Autodesk Fusion 360 part; units mm, degrees
(part 2 of 2)
sketch "Sketch1" plane through (0, 0, 0) normal (0, 0, 1) x (1, 0, 0)
  line L0 (8.5, 0) -> (91.5, 0)
  line L1 (100, 8.5) -> (100, 91.5)
  line L2 (91.5, 100) -> (8.5, 100)
  line L3 (0, 91.5) -> (0, 8.5)
  line L4 (8.5, 100) -> (8.5, 91.5)
  line L5 (8.5, 91.5) -> (0, 91.5)
  line L6 (91.5, 100) -> (91.5, 91.5)
  line L7 (91.5, 91.5) -> (100, 91.5)
  line L8 (8.5, 0) -> (8.5, 8.5)
  line L9 (8.5, 8.5) -> (0, 8.5)
  line L10 (91.5, 0) -> (91.5, 8.5)
  line L11 (91.5, 8.5) -> (100, 8.5)
  circle A0 centre (28.5, 95.75) radius 1.465
  circle A1 centre (71.5, 95.75) radius 1.465
  circle A2 centre (28.5, 4.25) radius 1.465
  circle A3 centre (71.5, 4.25) radius 1.465
  dimension "d11" = 8.5
  dimension "d12" = 8.5
  dimension "d13" = 8.5
  dimension "d14" = 8.5
  dimension "d15" = 8.5
  dimension "d16" = 8.5
  dimension "d17" = 83
  dimension "d18" = 83
  dimension "d19" = 8.5
  dimension "d20" = 8.5
  dimension "d21" = 8.5
  dimension "d22" = 8.5
  dimension "d25" = 2.93
  dimension "d26" = 4.25
  dimension "d27" = 20
  dimension "d28" = 2.93
  dimension "d29" = 4.25
  dimension "d30" = 20
  dimension "d31" = 2.93
  dimension "d32" = 4.25
  dimension "d33" = 20
  dimension "d34" = 2.93
  dimension "d35" = 4.25
  dimension "d36" = 20
  constraint horizontal L0
  constraint vertical L1
  constraint horizontal L2
  constraint vertical L3
  constraint vertical L4
  constraint horizontal L5
  constraint vertical L6
  constraint horizontal L7
  constraint vertical L8
  constraint horizontal L9
  constraint vertical L10
  constraint horizontal L11
  measures "d11" distance of L10.end L1.start
  measures "d12" distance of L0.end L10.end
  measures "d13" distance of L2.start L6.end
  measures "d14" distance of L6.end L1.end
  measures "d15" distance of L2.end L4.end
  measures "d16" distance of L4.end L3.start
  measures "d17" distance of L3.start L3.end
  measures "d18" distance of L0.start L0.end
  measures "d19" distance of L0.start L8.end
  measures "d20" distance of L8.end L3.end
  measures "d21" distance of origin L0.start
  measures "d22" distance of origin L9
  measures "d25" diameter of A0
  measures "d26" distance of L2 A0.centre
  measures "d27" distance of L4 A0.centre
  measures "d28" diameter of A1
  measures "d29" distance of L2 A1.centre
  measures "d30" distance of L6 A1.centre
  measures "d31" diameter of A2
  measures "d32" distance of L0 A2.centre
  measures "d33" distance of L8 A2.centre
  measures "d34" diameter of A3
  measures "d35" distance of L0 A3.centre
  measures "d36" distance of L10 A3.centre
extrude "Extrude1" add sketch "Sketch1" along normal blind 2

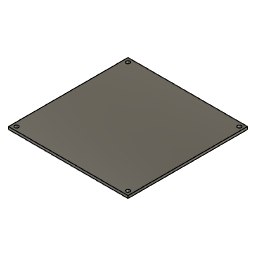
design "подставка"
Autodesk Fusion 360 part; units mm, degrees
sketch "Sketch1" plane through (0, 0, 0) normal (0, 0, 1) x (1, 0, 0)
  line L0 (0, 0) -> (96, 0)
  line L1 (96, 0) -> (96, 96)
  line L2 (96, 96) -> (0, 96)
  line L3 (0, 96) -> (0, 0)
  dimension "d1" = 96
  dimension "d2" = 96
  constraint horizontal L0
  constraint vertical L1
  constraint horizontal L2
  constraint vertical L3
  constraint coincident L0.start L3.end
  measures "d1" distance of L0.start L0.end
  measures "d2" distance of L0.start L2.end
extrude "Extrude1" add sketch "Sketch1" along normal blind 2
sketch "Sketch2" plane through (0, 0, 2) normal (0, 0, 1) x (-1, 0, 0)
  line L0 (0, -96) -> (0, 0)
  line L1 (0, 0) -> (-96, 0)
  line L2 (-96, 0) -> (-96, -96)
  line L3 (-96, -96) -> (0, -96)
  circle A0 centre (-3.25, -3.25) radius 1.5
  circle A1 centre (-3.25, -92.75) radius 1.5
  circle A2 centre (-92.75, -92.75) radius 1.5
  circle A3 centre (-92.75, -3.25) radius 1.5
  dimension "d5" = 3
  dimension "d6" = 3.25
  dimension "d7" = 3.25
  dimension "d8" = 3
  dimension "d9" = 3.25
  dimension "d10" = 3.25
  dimension "d11" = 3
  dimension "d12" = 3.25
  dimension "d13" = 3.25
  dimension "d14" = 3
  dimension "d15" = 3.25
  dimension "d16" = 3.25
  measures "d5" diameter of A0
  measures "d6" distance of L0 A0.centre
  measures "d7" distance of L1 A0.centre
  measures "d8" diameter of A1
  measures "d9" distance of L0 A1.centre
  measures "d10" distance of L3 A1.centre
  measures "d11" diameter of A2
  measures "d12" distance of L2 A2.centre
  measures "d13" distance of L3 A2.centre
  measures "d14" diameter of A3
  measures "d15" distance of L1 A3.centre
  measures "d16" distance of L2 A3.centre
extrude "Extrude2" cut sketch "Sketch2" against normal blind 2 contours A0 | A1 | A2 | A3

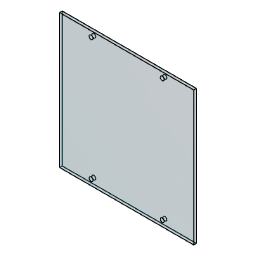
design "стенка2"
Autodesk Fusion 360 part; units mm, degrees
sketch "Sketch1" plane through (0, 0, 0) normal (0, 1, 0) x (1, 0, 0)
  line L0 (0, 0) -> (100, 0)
  line L1 (100, 0) -> (100, -100)
  line L2 (100, -100) -> (0, -100)
  line L3 (0, -100) -> (0, 0)
  circle A0 centre (23.5, -4.25) radius 1.465
  circle A1 centre (76.5, -4.25) radius 1.465
  circle A2 centre (23.5, -95.75) radius 1.465
  circle A3 centre (76.5, -95.75) radius 1.465
  dimension "d1" = 100
  dimension "d2" = 100
  dimension "d5" = 2.93
  dimension "d6" = 4.25
  dimension "d7" = 23.5
  dimension "d8" = 2.93
  dimension "d9" = 4.25
  dimension "d10" = 23.5
  dimension "d11" = 2.93
  dimension "d12" = 2.93
  dimension "d13" = 4.25
  dimension "d14" = 4.25
  dimension "d15" = 23.5
  dimension "d16" = 23.5
  constraint horizontal L0
  constraint vertical L1
  constraint horizontal L2
  constraint vertical L3
  constraint coincident L0.start L3.end
  measures "d1" distance of L0.start L0.end
  measures "d2" distance of L0.start L2.end
  measures "d5" diameter of A0
  measures "d6" distance of L0 A0.centre
  measures "d7" distance of L3 A0.centre
  measures "d8" diameter of A1
  measures "d9" distance of L0 A1.centre
  measures "d10" distance of L1 A1.centre
  measures "d11" diameter of A2
  measures "d12" diameter of A3
  measures "d13" distance of L2 A2.centre
  measures "d14" distance of L2 A3.centre
  measures "d15" distance of L3 A2.centre
  measures "d16" distance of L1 A3.centre
extrude "Extrude1" add sketch "Sketch1" along normal blind 2
